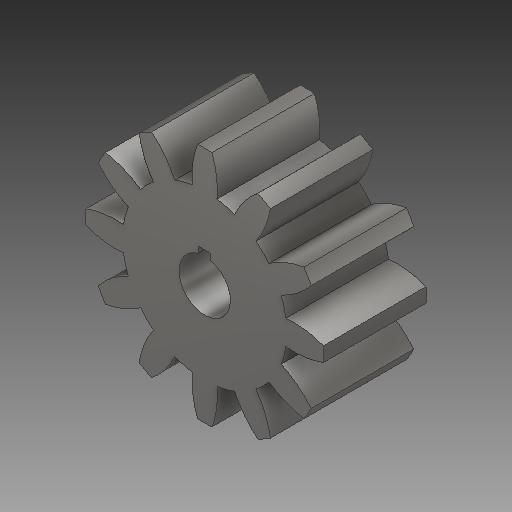
# Autodesk Inventor part: Gear
Saved by Autodesk Inventor 2018 (Build 220112000, 112)
## iProperties
Created: 2017-12-22
Part Number: Gear
Material: Stainless Steel
Document SubType Name: Modeling
Designer: 232963
Density: 8 g/cm^3
Appearance: Semi-Polished
Mass: 45.1261 g
Surface Area: 32.232 cm^2
Volume: 5.64076 cm^3
Author: 232963
Autodesk Inventor part; units mm, degrees
ref_plane "YZ Plane" through (0, 0, 0) normal (1, 0, 0) x (0, 1, 0)
ref_plane "XZ Plane" through (0, 0, 0) normal (0, 1, 0) x (-1, 0, 0)
ref_plane "XY Plane" through (0, 0, 0) normal (0, 0, 1) x (1, 0, 0)
sketch "Sketch1" plane through (0, 0, 0) normal (0, 0, 1) x (1, 0, 0)
  circle A0 centre (0, 0) radius 10.16
  arc A1 (-0.762, 3.0822) -> (0.762, 3.0822) centre (0, 0) ccw
  line L0 (0.762, 3.0822) -> (0.762, 3.8442)
  line L1 (0.762, 3.8442) -> (-0.762, 3.8442)
  line L2 (-0.762, 3.8442) -> (-0.762, 3.0822)
  point P0 (0, 3.0822)
  constraints: 6 end point, 2 centre point, 2 coincident, 2 point on circle, 1 parallel, 1 vertical alignment
extrude "Extrusion1" add sketch "Sketch1" along normal blind 12.7
sketch "Sketch2" plane through (0, 0, 12.7) normal (0, 0, 1) x (1, 0, 0)
  arc A0 (0.8854, 14.7054) -> (-0.8926, 14.7049) centre (0, 0) ccw
  arc A1 (-0.762, 3.0822) -> (0.762, 3.0822) centre (0, 0) ccw projected
  circle A2 centre (0, 0) radius 10.16 projected
  arc A3 (1.5168, 10.0461) -> (0.8854, 14.7054) centre (-8.8522, 11.0133) ccw
  arc A4 (-0.8926, 14.7049) -> (-1.524, 10.045) centre (8.8449, 11.0129) ccw
  dimension "d6" = 29.464
  dimension "d8" = 10.414
  dimension "d9" = 10.414
  dimension "d12" = 1.778
  constraints: 8 point on circle, 3 centre point, 1 coincident
  measures "d6" diameter of A0
  measures "d8" radius of A3
  measures "d9" radius of A4
  measures "d12" distance of A0.end A0.start
extrude "Extrusion2" add sketch "Sketch2" against normal blind 12.7 contours A3 A2 A4 A0
pattern_circular "Circular Pattern1" count 12 over 360 about axis through (0, 0, 0) along (0, 0, 1) of "Extrusion2"
body "Solid1"
